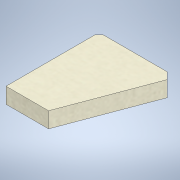
# Autodesk Inventor part: StrategyCard_All
Saved by Autodesk Inventor 2021 (Build 250183000, 183)
## iProperties
Created: 2023-03-16
Part Number: StrategyCard_All
Material: Paper
Document SubType Name: Modeling
Designer: Bradley
Density: 0.93 g/cm^3
Appearance: Cardboard - Chipboard
Author: Bradley
Autodesk Inventor part; units mm, degrees
ref_plane "YZ Plane" through (0, 0, 0) normal (1, 0, 0) x (0, 1, 0)
ref_plane "XZ Plane" through (0, 0, 0) normal (0, 1, 0) x (-1, 0, 0)
ref_plane "XY Plane" through (0, 0, 0) normal (0, 0, 1) x (1, 0, 0)
sketch "Sketch1" plane through (0, 0, 0) normal (0, 1, 0) x (-1, 0, 0)
  line L0 (31.575, 38.95) -> (-5.625, 38.95)
  line L1 (-5.625, 38.95) -> (-33.925, -36.6)
  line L2 (-33.925, -36.6) -> (-28.075, -42.45)
  line L3 (-28.075, -42.45) -> (28.075, -42.45)
  line L4 (28.075, -42.45) -> (31.575, -38.95)
  line L5 (31.575, -38.95) -> (31.575, 38.95)
  point P0 (0, 0)
  point P1 (0, -42.45)
  point P2 (31.575, 0)
  dimension "d0" = 3.5
  dimension "d1" = 3.5
  dimension "d2" = 81.4
  dimension "d3" = 37.2
  dimension "d4" = 65.5
  dimension "d5" = 59.65
  constraints: 12 end point, 3 perpendicular, 2 midpoint, 1 horizontal, 1 horizontal alignment, 1 vertical alignment
  measures "d0" horizontal distance of L3.end L4.end
  measures "d1" horizontal distance of L3.end L4.end
  measures "d2" distance between parallel lines of L0 L3
  measures "d3" distance of L0.start L0.end
  measures "d4" distance from line of L1.end L5
  measures "d5" distance from line of L5 L2.end
extrude "Extrusion1" add sketch "Sketch1" along normal mid plane 13.7
equation "\"d1\" = d0"
body "Solid1"
